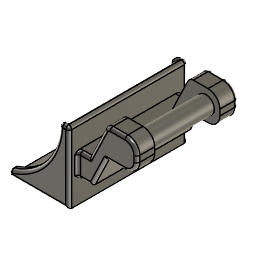
Dozer (Autodesk Fusion 360 design; units mm, degrees)
part number: 2026-03-22-23-28-42-444
Autodesk Fusion 360 part; units mm, degrees
note: some values were not read from the file. Set by a fixed rule: which face or edge a step refers to.
sketch "Sketch1" plane through (0, 0, 0) normal (0, 1, 0) x (1, 0, 0)
  line L0 (-25.4, 0) -> (0, 0)
  line L1 (0, 0) -> (0, -30.48)
  line L2 (0, -30.48) -> (-2.54, -30.48)
  arc A0 (-2.54, -30.48) -> (-25.4, 0) centre (-33.6513, -30.001) ccw
  dimension "d1" = 30.48
  dimension "d2" = 2.54
  dimension "d5" = 25.4
  dimension "d6" = 31.115
  constraint coincident L0.end L1.start
  constraint horizontal L0
  constraint perpendicular L0 L1
  constraint perpendicular L1 L2
  constraint coincident L0.start A0.end
  measures "d1" distance of L0.end L1.end
  measures "d2" distance of L1.end L2.end
  measures "d5" distance of L0.start L0.end
  measures "d6" radius of A0
extrude "Extrude1" add sketch "Sketch1" along normal mid plane 50.8
sketch "Sketch2" plane through (0, 0, 0) normal (1, 0, 0) x (0, 1, 0)
  line L0 (-25.4, 0) -> (25.4, 0)
  line L1 (25.4, 0) -> (25.4, 30.48)
  line L2 (25.4, 30.48) -> (-25.4, 30.48)
  line L3 (-25.4, 30.48) -> (-25.4, 0)
  line L4 (-13.97, 20.32) -> (13.97, 20.32)
  line L5 (13.97, 20.32) -> (13.97, 10.16)
  line L6 (13.97, 10.16) -> (-13.97, 10.16)
  line L7 (-13.97, 10.16) -> (-13.97, 20.32)
  dimension "d9" = 27.94
  dimension "d10" = 10.16
  dimension "d11" = 10.16
  dimension "d12" = 11.43
  constraint horizontal L4
  constraint vertical L5
  constraint horizontal L6
  constraint vertical L7
  measures "d9" distance of L4.start L4.end
  measures "d10" distance of L4.start L6.end
  measures "d11" distance of L0 L6
  measures "d12" distance of L3 L7
extrude "Extrude2" add sketch "Sketch2" along normal blind 10.16 contours L4 L5 L6 L7
sketch "Sketch3" plane through (0, -13.97, 0) normal (0, -1, 0) x (1, 0, 0)
  line L0 (0, 20.32) -> (0, 10.16)
  line L1 (0, 10.16) -> (10.16, 10.16)
  line L2 (10.16, 10.16) -> (10.16, 20.32)
  line L3 (10.16, 20.32) -> (0, 20.32)
  line L4 (5.08, 20.32) -> (12.4091, 35.56)
  line L5 (12.4091, 35.56) -> (25.4, 35.56)
  line L6 (25.4, 35.56) -> (25.4, 22.86)
  line L7 (25.4, 22.86) -> (12.4576, 22.86)
  line L8 (12.4576, 22.86) -> (6.35, 10.16)
  line L9 (5.08, 20.32) -> (0, 20.32)
  line L10 (0, 10.16) -> (6.35, 10.16)
  line L11 (0, 20.32) -> (0, 10.16)
  line L12 (-25.4, 0) -> (0, 0)
  dimension "d22" = 25.4
  dimension "d23" = 22.86
  dimension "d24" = 12.7
  constraint perpendicular L0 L5
  constraint perpendicular L5 L6
  constraint perpendicular L6 L7
  constraint parallel L4 L8
  constraint midpoint L3 L4.start
  constraint coincident L0.start L3.end
  constraint coincident L0.end L1.start
  constraint perpendicular L0 L10
  measures "d22" distance of L6 L11
  measures "d23" distance of L7 L12
  measures "d24" distance of L5 L7
extrude "Extrude3" add sketch "Sketch3" along normal blind 7.62 contours L0 L1 L2 L3 L8 L9 L10 L11 | L2 L3 L4 L5 L6 L7 L8
mirror "Mirror1" about plane through (0, 0, 0) normal (0, 1, 0) of "Extrude3"
sketch "Sketch4" plane through (0, -13.97, 0) normal (0, 1, 0) x (-1, 0, 0)
  line L0 (-10.16, 20.32) -> (-5.08, 20.32)
  line L1 (-5.08, 20.32) -> (-12.4091, 35.56)
  line L2 (-12.4091, 35.56) -> (-25.4, 35.56)
  line L3 (-25.4, 35.56) -> (-25.4, 22.86)
  line L4 (-25.4, 22.86) -> (-12.4576, 22.86)
  line L5 (-12.4576, 22.86) -> (-10.16, 18.0824)
  line L6 (-10.16, 18.0824) -> (-10.16, 20.32)
  circle A0 centre (-19.346, 29.21) radius 3.683
  line L7 (-32.4673, 29.21) -> (-5.1482, 29.21) construction
  dimension "d19" = 7.366
  constraint perpendicular L3 L7
  constraint coincident A0.centre L7
  measures "d19" diameter of A0
extrude "Extrude4" add sketch "Sketch4" along normal up to surface (27.94 mm away) contours A0
extrude "Extrude5" cut 1 faces at (8.89, -13.97, 12.8008) along direction (0, 1, 0) through all
sketch "Sketch5" plane through (0, -25.4, 0) normal (0, -1, 0) x (1, 0, 0)
  line L0 (0, 30.48) -> (-2.54, 30.48)
  arc A0 (-25.4, 0) -> (-2.54, 30.48) centre (-33.6513, 30.001) ccw
  line L1 (-25.4, 0) -> (0, 0)
  line L2 (0, 0) -> (0, 30.48)
  line L3 (0, 0) -> (-25.4, 0)
  line L4 (-25.4, 0) -> (-25.4, 2.54)
  line L5 (0, 0) -> (0, 30.48)
  line L6 (0, 30.48) -> (-3.81, 30.48)
  arc A1 (-25.4, 2.54) -> (-3.81, 30.48) centre (-33.6723, 31.2438) ccw
  constraint coincident L1.end L2.start
  constraint coincident A0.start L1.start
  constraint perpendicular L3 L4
  constraint coincident L0.start L2.end
  constraint perpendicular L2 L6
  constraint tangent A0 A1
extrude "Extrude6" add sketch "Sketch5" against normal blind 2.54
mirror "Mirror2" about plane through (0, 0, 0) normal (0, 1, 0) of "Extrude6"
fillet "Fillet1" radius 1.27 2 edges at (-25.4, -24.13, 2.54) (-25.4, 24.13, 2.54) 3 faces at (-0.8467, -7.62, 30.48) (-1.7311, -25.4, 17.5693) (-1.7311, 25.4, 17.5693)
fillet "Fillet2" radius 1.27 2 faces at (16.7556, 21.59, 31.3267) (16.7556, -21.59, 31.3267)
fillet "Fillet3" radius 5.08 8 edges at (25.4, -17.145, 35.56) (25.028, -21.218, 35.188) (25.4, -17.145, 22.86) (25.028, -21.218, 23.232) (25.4, 17.145, 22.86) (25.028, 21.218, 23.232) (25.4, 17.145, 35.56) (25.028, 21.218, 35.188)
fillet "Fillet4" radius 2.54 4 edges at (12.4091, 17.145, 35.56) (12.643, 21.218, 35.188) (12.4091, -17.145, 35.56) (12.643, -21.218, 35.188)
